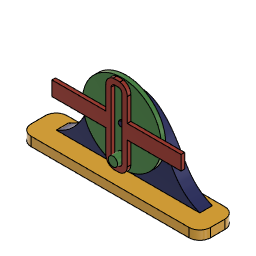
Scotch-Yoke (Autodesk Fusion 360 design; units mm, degrees)
Autodesk Fusion 360 part; units mm, degrees
note: some values were not read from the file. Set by a fixed rule: which sketch regions a step uses.
sketch "Baza" plane through (0, 0, 0) normal (0, 0, 1) x (1, 0, 0) in component "Baza"
  line L0 (-22, 5) -> (22, 5)
  line L1 (25, 2) -> (25, -2)
  line L2 (22, -5) -> (-22, -5)
  line L3 (-25, -2) -> (-25, 2)
  arc A0 (25, 2) -> (22, 5) centre (22, 2) ccw
  arc A1 (22, -5) -> (25, -2) centre (22, -2) ccw
  arc A2 (-22, 5) -> (-25, 2) centre (-22, 2) ccw
  arc A3 (-25, -2) -> (-22, -5) centre (-22, -2) ccw
  dimension "d1" = 3
  constraint horizontal L0
  constraint vertical L1
  constraint horizontal L2
  constraint vertical L3
  constraint tangent L0 A0
  constraint tangent L1 A0
  constraint tangent L1 A1
  constraint tangent L2 A1
  constraint equal A0 A1
  constraint tangent L0 A2
  constraint tangent L3 A2
  constraint equal A0 A2
  constraint tangent L2 A3
  constraint tangent L3 A3
  constraint equal A0 A3
  measures "d1" radius of A0
extrude "Extrude1" add sketch "Baza" along normal blind 2.5 makes body 1 in component "Baza"
sketch "Holder" plane through (0, 0, 0) normal (0, 1, 0) x (1, 0, 0) in component "Holder"
  spline S0 degree 5 poles (-20, -2.5) (-19.6612, -2.6375) (-19.0005, -2.9259) (-18.0603, -3.3988) (-16.9085, -4.1099) (-15.6352, -5.1338) (-14.5158, -6.2929) (-13.5252, -7.5863) (-12.6179, -9.0121) (-11.7308, -10.5642) (-10.7949, -12.2255) (-9.7452, -13.962) (-8.5307, -15.7171) (-7.1261, -17.4027) (-5.5361, -18.9027) (-3.7875, -20.0942) (-1.9239, -20.8653) (0, -21.1336) (1.9239, -20.8653) (3.7875, -20.0942) (5.5361, -18.9027) (7.1261, -17.4027) (8.5307, -15.7171) (9.7452, -13.962) (10.7949, -12.2255) (11.7308, -10.5642) (12.6179, -9.0121) (13.5252, -7.5863) (14.5158, -6.2929) (15.6352, -5.1338) (16.9085, -4.1099) (18.0603, -3.3988) (19.0005, -2.9259) (19.6612, -2.6375) (20, -2.5) knots 0 0 0 0 0 0 0.033333 0.066667 0.1 0.133333 0.166667 0.2 0.233333 0.266667 0.3 0.333333 0.366667 0.4 0.433333 0.466667 0.5 0.533333 0.566667 0.6 0.633333 0.666667 0.7 0.733333 0.766667 0.8 0.833333 0.866667 0.9 0.933333 0.966667 1 1 1 1 1 1
  line L0 (-20, -2.5) -> (20, -2.5)
  point P0 (-14, -7)
  point P1 (-9, -15)
  point P2 (0, -21)
  point P3 (9, -15)
  point P4 (14, -7)
  constraint horizontal L0
extrude "Extrude1'" add sketch "Holder" along normal blind 3.5 separate body makes body 2 in component "Holder"
sketch "Joint_baza" plane through (0, 0, 0) normal (0, 0, 1) x (1, 0, 0) in component "Holder"
  line L0 (-5, 0) -> (5, 0)
  line L1 (5, 0) -> (5, 3.5)
  line L2 (5, 3.5) -> (-5, 3.5)
  line L3 (-5, 3.5) -> (-5, 0)
  constraint horizontal L0
  constraint perpendicular L0 L1
  constraint perpendicular L1 L2
  constraint perpendicular L0 L3
extrude "Extrude2" add sketch "Joint_baza" along normal blind 2.5 bodies 2 in component "Holder"
extrude "Extrude2'" cut sketch "Joint_baza" along normal blind 2.5 bodies 1 in component "Baza"
extrude "Extrude4" add sketch "Joint_baza" along normal blind 2.5 bodies 2 in component "Holder"
sketch "Joint_cerc" plane through (0, 0, 0) normal (0, -1, 0) x (1, 0, 0) in component "Holder"
  line L0 (-20, 2.5) -> (-5, 2.5)
  line L1 (-5, 2.5) -> (-5, 0)
  line L2 (-5, 0) -> (5, 0)
  line L3 (5, 0) -> (5, 2.5)
  line L4 (5, 2.5) -> (20, 2.5)
  spline S0 degree 5 poles (-20, 2.5) (-19.6612, 2.6375) (-19.0005, 2.9259) (-18.0603, 3.3988) (-16.9085, 4.1099) (-15.6352, 5.1338) (-14.5158, 6.2929) (-13.5252, 7.5863) (-12.6179, 9.0121) (-11.7308, 10.5642) (-10.7949, 12.2255) (-9.7452, 13.962) (-8.5307, 15.7171) (-7.1261, 17.4027) (-5.5361, 18.9027) (-3.7875, 20.0942) (-1.9239, 20.8653) (0, 21.1336) (1.9239, 20.8653) (3.7875, 20.0942) (5.5361, 18.9027) (7.1261, 17.4027) (8.5307, 15.7171) (9.7452, 13.962) (10.7949, 12.2255) (11.7308, 10.5642) (12.6179, 9.0121) (13.5252, 7.5863) (14.5158, 6.2929) (15.6352, 5.1338) (16.9085, 4.1099) (18.0603, 3.3988) (19.0005, 2.9259) (19.6612, 2.6375) (20, 2.5) knots 0 0 0 0 0 0 0.033333 0.066667 0.1 0.133333 0.166667 0.2 0.233333 0.266667 0.3 0.333333 0.366667 0.4 0.433333 0.466667 0.5 0.533333 0.566667 0.6 0.633333 0.666667 0.7 0.733333 0.766667 0.8 0.833333 0.866667 0.9 0.933333 0.966667 1 1 1 1 1 1
  circle A0 centre (0, 15) radius 0.7
extrude "Extrude5" add sketch "Joint_cerc" along normal blind 2 contours A0 bodies 2 in component "Holder"
sketch "Cerc" plane through (0, 0, 0) normal (0, -1, 0) x (1, 0, 0) in component "Cerc"
  circle A0 centre (0, 15) radius 0.7
  line L0 (-20, 2.5) -> (-5, 2.5)
  line L1 (-5, 2.5) -> (-5, 0)
  line L2 (-5, 0) -> (5, 0)
  line L3 (5, 0) -> (5, 2.5)
  line L4 (5, 2.5) -> (20, 2.5)
  spline S0 degree 5 poles (-20, 2.5) (-19.6612, 2.6375) (-19.0005, 2.9259) (-18.0603, 3.3988) (-16.9085, 4.1099) (-15.6352, 5.1338) (-14.5158, 6.2929) (-13.5252, 7.5863) (-12.6179, 9.0121) (-11.7308, 10.5642) (-10.7949, 12.2255) (-9.7452, 13.962) (-8.5307, 15.7171) (-7.1261, 17.4027) (-5.5361, 18.9027) (-3.7875, 20.0942) (-1.9239, 20.8653) (0, 21.1336) (1.9239, 20.8653) (3.7875, 20.0942) (5.5361, 18.9027) (7.1261, 17.4027) (8.5307, 15.7171) (9.7452, 13.962) (10.7949, 12.2255) (11.7308, 10.5642) (12.6179, 9.0121) (13.5252, 7.5863) (14.5158, 6.2929) (15.6352, 5.1338) (16.9085, 4.1099) (18.0603, 3.3988) (19.0005, 2.9259) (19.6612, 2.6375) (20, 2.5) knots 0 0 0 0 0 0 0.033333 0.066667 0.1 0.133333 0.166667 0.2 0.233333 0.266667 0.3 0.333333 0.366667 0.4 0.433333 0.466667 0.5 0.533333 0.566667 0.6 0.633333 0.666667 0.7 0.733333 0.766667 0.8 0.833333 0.866667 0.9 0.933333 0.966667 1 1 1 1 1 1
  circle A1 centre (0, 15) radius 11
  circle A2 centre (0, 15) radius 0.8
  constraint concentric A0 A1
  constraint concentric A1 A2
extrude "Extrude1''" add sketch "Cerc" along normal blind 1.2 separate body contours S0 A1 | S0 A1 makes body 3 in component "Cerc"
move_body "Move1" bodies 3 to x (1, 0, 0) y (0, 1, 0) z (0, 0, 1) at (0, -0.6, 0) in component "Cerc"
sketch "Bump" plane through (0, -1.8, 0) normal (0, -1, 0) x (1, 0, 0) in component "Cerc"
  circle A0 centre (0, 15) radius 0.8
  circle A1 centre (0, 15) radius 11
  circle A2 centre (0, 7) radius 1.3
extrude "Extrude2''" add sketch "Bump" along normal blind 2.5 contours A2 bodies 3 in component "Cerc"
sketch "Circle_mover" plane through (0, -1.8, 0) normal (0, -1, 0) x (1, 0, 0) in component "Bar_slide"
  circle A0 centre (0, 7) radius 1.3
  circle A1 centre (0, 15) radius 0.8
  circle A2 centre (0, 15) radius 11
  line L0 (-0.5, 5.5) -> (0.5, 5.5)
  line L1 (1.5, 6.5) -> (1.5, 23.5)
  line L2 (0.5, 24.5) -> (-0.5, 24.5)
  line L3 (-1.5, 23.5) -> (-1.5, 6.5)
  arc A3 (-1.5, 6.5) -> (-0.5, 5.5) centre (-0.5, 6.5) ccw
  arc A4 (0.5, 5.5) -> (1.5, 6.5) centre (0.5, 6.5) ccw
  arc A5 (-0.5, 24.5) -> (-1.5, 23.5) centre (-0.5, 23.5) ccw
  arc A6 (1.5, 23.5) -> (0.5, 24.5) centre (0.5, 23.5) ccw
  line L4 (-0.5, 4) -> (0.5, 4)
  arc A7 (0.5, 4) -> (3, 6.5) centre (0.5, 6.5) ccw
  line L5 (3, 6.5) -> (3, 23.5)
  arc A8 (3, 23.5) -> (0.5, 26) centre (0.5, 23.5) ccw
  line L6 (0.5, 26) -> (-0.5, 26)
  arc A9 (-0.5, 26) -> (-3, 23.5) centre (-0.5, 23.5) ccw
  line L7 (-3, 23.5) -> (-3, 6.5)
  arc A10 (-3, 6.5) -> (-0.5, 4) centre (-0.5, 6.5) ccw
  dimension "d20" = 1
  dimension "d21" = 1.5
  constraint horizontal L0
  constraint perpendicular L0 L1
  constraint perpendicular L1 L2
  constraint perpendicular L0 L3
  constraint tangent L0 A3
  constraint tangent L3 A3
  constraint tangent L0 A4
  constraint tangent L1 A4
  constraint equal A3 A4
  constraint tangent L2 A5
  constraint tangent L3 A5
  constraint equal A3 A5
  constraint tangent L1 A6
  constraint tangent L2 A6
  constraint equal A3 A6
  measures "d20" radius of A3
extrude "Extrude1'''" add sketch "Circle_mover" along normal blind 1 separate body contours A2 A7 L5 A8 A9 L7 A10 makes body 4 in component "Bar_slide"
move_body "Move1'" bodies 4 to x (1, 0, 0) y (0, 1, 0) z (0, 0, 1) at (0, -0.8, 0) in component "Bar_slide"
sketch "Piston_R" plane through (3, 0, 0) normal (1, 0, 0) x (0, 1, 0) in component "Bar_slide"
  line L0 (-2.6, 6.5) -> (-2.6, 23.5)
  line L1 (-2.6, 23.5) -> (-3.6, 23.5)
  line L2 (-3.6, 23.5) -> (-3.6, 6.5)
  line L3 (-3.6, 6.5) -> (-2.6, 6.5)
  line L4 (-3.6, 17.0002) -> (-2.6, 17.0002)
  line L5 (-2.6, 17.0002) -> (-2.6, 13.0027)
  line L6 (-2.6, 13.0027) -> (-3.6, 13.0027)
  line L7 (-3.6, 17.0002) -> (-3.6, 13.0027)
  constraint coincident L2 L4.start
  constraint coincident L0 L4.end
  constraint perpendicular L0 L4
  constraint coincident L0 L5.end
  constraint coincident L2 L6.end
  constraint perpendicular L2 L6
sketch "Piston_L" plane through (-3, 0, 0) normal (-1, 0, 0) x (0, -1, 0) in component "Bar_slide"
  line L0 (2.6, 23.5) -> (2.6, 6.5)
  line L1 (2.6, 6.5) -> (3.6, 6.5)
  line L2 (3.6, 6.5) -> (3.6, 23.5)
  line L3 (3.6, 23.5) -> (2.6, 23.5)
  line L4 (2.6, 17.0004) -> (3.6, 17.0004)
  line L5 (3.6, 17.0004) -> (3.6, 12.9969)
  line L6 (3.6, 12.9969) -> (2.6, 12.9969)
  line L7 (2.6, 12.9969) -> (2.6, 17.0004)
  constraint coincident L0 L4.start
  constraint coincident L2 L4.end
  constraint perpendicular L2 L4
  constraint coincident L2 L5.end
  constraint coincident L0 L6.end
  constraint perpendicular L0 L6
extrude "Extrude2'''" add sketch "Piston_R" along normal blind 15 contours L0 L2 L4 L5 L6 L7 bodies 4 in component "Bar_slide"
extrude "Extrude3" add sketch "Piston_L" along normal blind 15 contours L0 L2 L4 L5 L6 L7 bodies 4 in component "Bar_slide"
component "Baza" placed x (1, 0, 0) y (0, 1, 0) z (0, 0, 1) at (0, 0, 0)
component "Holder" placed x (1, 0, 0) y (0, 1, 0) z (0, 0, 1) at (0, 0, 0)
component "Cerc" placed x (1, 0, 0) y (0, 1, 0) z (0, 0, 1) at (0, 0.1, 0)
component "Bar_slide" placed x (1, 0, 0) y (0, -1, 0) z (0, 0, -1) at (0, -5.6, 30)
named bodies: "Baza", "Holder", "Cerc", "Slide"
